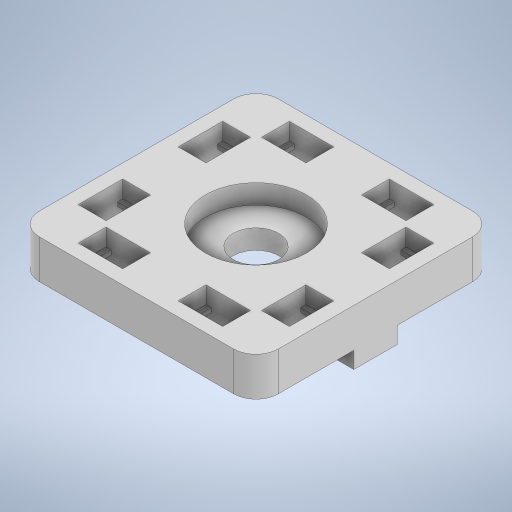
# Autodesk Inventor part: SigmaSideConnection
Saved by Autodesk Inventor 2024 (Build 280153000, 153)
## iProperties
Created: 2024-04-07
Part Number: SigmaSideConnection
Material: Generic
Document SubType Name: Modeling
Designer: Admin
Density: 1 g/cm^3
Appearance: Default
Author: Admin
Autodesk Inventor part; units mm, degrees
ref_plane "YZ Plane" through (0, 0, 0) normal (1, 0, 0) x (0, 1, 0)
ref_plane "XZ Plane" through (0, 0, 0) normal (0, 1, 0) x (-1, 0, 0)
ref_plane "XY Plane" through (0, 0, 0) normal (0, 0, 1) x (1, 0, 0)
sketch "Sketch1" plane through (0, 0, 0) normal (0, 1, 0) x (-1, 0, 0)
  line L0 (0, 0) -> (43, 0)
  line L1 (43, 0) -> (43, -43)
  line L2 (43, -43) -> (0, -43)
  line L3 (0, -43) -> (0, 0)
  circle A0 centre (21.5, -21.5) radius 4.1
  line L4 (21.5, -43) -> (21.5, -21.5) construction
  line L5 (21.5, -21.5) -> (0, -21.5) construction
  line L6 (34.5, -35.5) -> (26.5, -35.5)
  line L7 (26.5, -35.5) -> (26.5, -40.5)
  line L8 (26.5, -40.5) -> (34.5, -40.5)
  line L9 (34.5, -40.5) -> (34.5, -35.5)
  line L10 (16.5, -35.5) -> (8.5, -35.5)
  line L11 (8.5, -35.5) -> (8.5, -40.5)
  line L12 (8.5, -40.5) -> (16.5, -40.5)
  line L13 (16.5, -40.5) -> (16.5, -35.5)
  line L14 (12.5, -35.5) -> (12.5, -40.5) construction
  line L15 (30.5, -35.5) -> (30.5, -40.5) construction
  line L16 (12.5, -38) -> (30.5, -38) construction
  line L17 (7.5, -34.5) -> (7.5, -26.5)
  line L18 (2.5, -34.5) -> (7.5, -34.5)
  line L19 (2.5, -26.5) -> (2.5, -34.5)
  line L20 (7.5, -26.5) -> (2.5, -26.5)
  line L21 (2.5, -16.5) -> (7.5, -16.5)
  line L22 (2.5, -8.5) -> (2.5, -16.5)
  line L23 (7.5, -16.5) -> (7.5, -8.5)
  line L24 (7.5, -8.5) -> (2.5, -8.5)
  line L25 (8.5, -7.5) -> (16.5, -7.5)
  line L26 (8.5, -2.5) -> (8.5, -7.5)
  line L27 (16.5, -2.5) -> (8.5, -2.5)
  line L28 (16.5, -7.5) -> (16.5, -2.5)
  line L29 (26.5, -2.5) -> (26.5, -7.5)
  line L30 (34.5, -2.5) -> (26.5, -2.5)
  line L31 (26.5, -7.5) -> (34.5, -7.5)
  line L32 (34.5, -7.5) -> (34.5, -2.5)
  line L33 (35.5, -8.5) -> (35.5, -16.5)
  line L34 (40.5, -8.5) -> (35.5, -8.5)
  line L35 (40.5, -16.5) -> (40.5, -8.5)
  line L36 (35.5, -16.5) -> (40.5, -16.5)
  line L37 (40.5, -26.5) -> (35.5, -26.5)
  line L38 (40.5, -34.5) -> (40.5, -26.5)
  line L39 (35.5, -26.5) -> (35.5, -34.5)
  line L40 (35.5, -34.5) -> (40.5, -34.5)
  point P0 (21.5, -38)
  point P1 (7.5, -30.5)
  point P2 (2.5, -30.5)
  point P3 (2.5, -12.5)
  point P4 (7.5, -12.5)
  point P5 (12.5, -7.5)
  point P6 (12.5, -2.5)
  point P7 (30.5, -2.5)
  point P8 (30.5, -7.5)
  point P9 (35.5, -12.5)
  point P10 (40.5, -12.5)
  point P11 (40.5, -30.5)
  point P12 (35.5, -30.5)
  dimension "d0" = 43
  dimension "d1" = 8.2
  dimension "d2" = 18
  dimension "d3" = 8
  dimension "d4" = 5
  dimension "d8" = 14
  dimension "d11" = 360
  constraints: 82 end point, 9 midpoint, 9 point on line, 6 parallel, 4 horizontal, 3 perpendicular, 2 equal length, 1 centre point, 1 vertical, 81 other
  measures "d0" distance between parallel lines of L3 L1
  measures "d1" diameter of A0
  measures "d2" distance of L16.start L16.end
  measures "d3" distance between parallel lines of L9 L7
  measures "d4" distance between parallel lines of L8 L6
  measures "d8" distance from line of L6 L4.end
extrude "Extrusion1" add sketch "Sketch1" along normal blind 7
sketch "Sketch3" plane through (-26.5, 0, -35.5) normal (0, 0, -1) x (-1, 0, 0)
  line L0 (0, 0) -> (0, 7) projected
  line L1 (0, 3.9) -> (0.9, 3.9)
  line L2 (0.9, 3.9) -> (0.9, 3.1)
  line L3 (0.9, 3.1) -> (0, 3.1)
  line L4 (0, 3.1) -> (0, 3.9)
  line L5 (8, 3.9) -> (7.1, 3.9)
  line L6 (7.1, 3.9) -> (7.1, 3.1)
  line L7 (7.1, 3.1) -> (8, 3.1)
  line L8 (8, 3.1) -> (8, 3.1)
  line L9 (0, 7) -> (8, 7) projected
  line L10 (8, 7) -> (8, 3.1)
  line L11 (8, 3.1) -> (8, 0.9742)
  line L12 (8, 3.1) -> (8, 3.9)
  line L13 (7.1, 3.5) -> (0.9, 3.5) construction
  line L14 (3.9585, 7) -> (3.9585, 0) construction
  line L15 (0, 0) -> (8, 0) projected
  point P0 (-26.5, 0)
  point P1 (3.9585, 3.5)
  point P2 (0, 3.1)
  dimension "d15" = 0.8
  dimension "d16" = 0.9
  constraints: 26 end point, 5 parallel, 5 point on line, 3 horizontal, 3 midpoint, 3 vertical, 2 collinear, 2 perpendicular
  measures "d15" distance between parallel lines of L5 L7
  measures "d16" distance between parallel lines of L10 L6
extrude "Extrusion2" add sketch "Sketch3" along normal up to surface (5 mm away)
sketch "Sketch4" plane through (-8.5, 0, -35.5) normal (0, 0, -1) x (-1, 0, 0)
  line L0 (8, 3.9) -> (7.1, 3.9)
  line L1 (7.1, 3.9) -> (7.1, 3.1)
  line L2 (7.1, 3.1) -> (8, 3.1)
  line L3 (8, 3.1) -> (8, 3.9)
  line L4 (0.9, 3.9) -> (0, 3.9)
  line L5 (0, 3.9) -> (0, 3.1)
  line L6 (0, 3.1) -> (0.9, 3.1)
  line L7 (0.9, 3.1) -> (0.9, 3.9)
  line L8 (0, 7) -> (8, 7) projected
  line L9 (3.7202, 7) -> (3.7202, 0) construction
  line L10 (0, 0) -> (8, 0) projected
  line L11 (7.1, 3.5) -> (3.7202, 3.5) construction
  line L12 (0.9, 3.5) -> (3.7202, 3.5) construction
  line L13 (0, 0) -> (0, 7) projected
  line L14 (8, 0) -> (8, 7) projected
  point P0 (-8.5, 0)
  dimension "d19" = 0.9
  dimension "d20" = 0.8
  constraints: 22 end point, 4 parallel, 3 collinear, 3 horizontal, 3 midpoint, 2 equal length, 2 perpendicular, 2 point on line, 1 vertical
  measures "d19" distance between parallel lines of L14 L1
  measures "d20" distance between parallel lines of L2 L0
extrude "Extrusion4" add sketch "Sketch4" along normal up to surface (5 mm away) contours L3 L2 L1 L0 | L4 L7 L6 L5
pattern_circular "Circular Pattern1" count 4 over 360 about axis through (-21.5, 0, -21.5) along (0, 1, 0) of "Extrusion4", "Extrusion2"
fillet "Fillet1" radius 4 4 edges at (-43, 3.5, -43) (-43, 3.5, 0) (0, 3.5, 0) (0, 3.5, -43)
sketch "Sketch6" plane through (0, 7, 0) normal (0, 1, 0) x (1, 0, 0)
  circle A0 centre (-21.5, 21.5) radius 4.1 projected
  circle A1 centre (-21.5, 21.5) radius 9.1
  point P0 (0, 0)
  dimension "d30" = 18.2
  constraints: 1 centre point, 1 coincident
  measures "d30" diameter of A1
extrude "Extrusion5" cut sketch "Sketch6" against normal blind 3.5
sketch "Sketch7" plane through (0, 0, 0) normal (0, -1, 0) x (1, 0, 0)
  line L0 (0, -4) -> (0, -39) projected
  line L1 (0, -17.6) -> (-10, -17.6)
  line L2 (-10, -17.6) -> (-10, -25.4)
  line L3 (-10, -25.4) -> (0, -25.4)
  line L4 (0, -25.4) -> (0, -17.6)
  line L5 (-43, -39) -> (-43, -4) projected
  line L6 (-33, -17.6) -> (-43, -17.6)
  line L7 (-43, -17.6) -> (-43, -25.4)
  line L8 (-43, -25.4) -> (-33, -25.4)
  line L9 (-33, -25.4) -> (-33, -17.6)
  line L10 (-10, -21.5) -> (-33, -21.5) construction
  circle A0 centre (-21.5, -21.5) radius 4.1 projected
  point P0 (0, 0)
  point P1 (0, -25.4)
  dimension "d33" = 7.8
  dimension "d34" = 10
  constraints: 18 end point, 4 parallel, 3 horizontal, 3 midpoint, 3 point on line, 2 perpendicular, 1 coincident, 1 collinear
  measures "d33" distance between parallel lines of L3 L1
  measures "d34" distance between parallel lines of L0 L2
extrude "Extrusion6" add sketch "Sketch7" along normal blind 3 contours L0 L3 L2 L1 | L5 L6 L9 L8
fillet "Fillet2" radius 2 4 edges at (-33, -1.5, -25.4) (-33, -1.5, -17.6) (-10, -1.5, -25.4) (-10, -1.5, -17.6)
body "Solid1"
